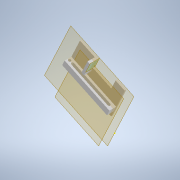
# Autodesk Inventor part: s_support_bottom
Saved by Autodesk Inventor 2020.1 (Build 241239000, 239)
## iProperties
Created: 2019-10-17
Part Number: s_support_bottom
Material: Generic
Document SubType Name: Modeling
Designer: jesse
Density: 1 g/cm^3
Appearance: Default
support_length: 2.300 in
hole_size: 0.118 in
Author: jesse
Autodesk Inventor part; units mm, degrees
ref_plane "YZ Plane" through (0, 0, 0) normal (1, 0, 0) x (0, 1, 0)
ref_plane "XZ Plane" through (0, 0, 0) normal (0, 1, 0) x (-1, 0, 0)
ref_plane "XY Plane" through (0, 0, 0) normal (0, 0, 1) x (1, 0, 0)
ref_plane "Work Plane1" through (19.722, 36.341, 0) normal (0, 0, 1) x (0.4250843, 0.9051538, 0)
sketch "Sketch1" plane through (19.722, 36.341, 0) normal (0, 0, 1) x (0.4250843, 0.9051538, 0)
  line L0 (-12.1227, 70.1452) -> (-18.8796, 70.1452)
  line L1 (-18.8796, 70.1452) -> (-18.8796, 11.7252)
  line L2 (-18.8796, 11.7252) -> (-12.1227, 11.7252)
  line L3 (-12.1227, 11.7252) -> (-12.1227, 70.1452)
  point P0 (-41.2777, 2.4034)
  dimension "support_length" = 58.42
  constraints: 8 end point, 2 parallel, 1 horizontal, 1 perpendicular
  measures "support_length" distance of L2.end L0.start
extrude "Extrusion1" add sketch "Sketch1" along normal blind 8
sketch "Sketch2" plane through (1.0834, 24.2363, 0) normal (-0.4250843, -0.9051538, 0) x (0, 0, 1)
  line L0 (0, 58.42) -> (8, 58.42) construction
  line L1 (4, 58.42) -> (4, 0) construction
  line L2 (0, 0) -> (8, 0) construction
  line L3 (4, 52.42) -> (4, 5) construction
  line L4 (2.5, 52.42) -> (2.5, 5)
  line L5 (5.5, 5) -> (5.5, 52.42)
  arc A0 (5.5, 52.42) -> (2.5, 52.42) centre (4, 52.42) ccw
  arc A1 (2.5, 5) -> (5.5, 5) centre (4, 5) ccw
  line L6 (4, 5) -> (6.3728, 5) construction
  line L7 (4, 52.42) -> (6.6371, 52.42) construction
  line L8 (5.634, 5) -> (5.634, 0) construction
  circle A2 centre (4, 56.42) radius 1.5
  line L9 (4, 56.42) -> (7.1435, 56.42) construction
  point P0 (0, -9.3218)
  point P1 (4, 28.71)
  dimension "d5" = 3
  dimension "d6" = 3
  dimension "d7" = 2
  dimension "d8" = 5
  dimension "d9" = 4
  constraints: 18 end point, 5 point on line, 4 point on circle, 4 tangent, 3 centre point, 3 horizontal, 3 midpoint, 1 parallel
  measures "d5" distance between parallel lines of L4 L5
  measures "d6" diameter of A2
  measures "d7" distance between parallel lines of L9 L0
  measures "d8" distance between parallel lines of L6 L2
  measures "d9" distance between parallel lines of L7 L9
extrude "Extrusion2" cut sketch "Sketch2" against normal blind 15.875
sketch "Sketch3" plane through (19.722, 36.341, 0) normal (0, 0, -1) x (-0.9051538, 0.4250843, 0)
  line L0 (70.1452, -12.1227) -> (70.1452, -18.8796) construction
  line L1 (11.7252, -12.1227) -> (70.1452, -12.1227) construction
  line L2 (70.1452, -18.8796) -> (11.7252, -12.1227) construction
  line L3 (70.1452, -4.7378) -> (11.7252, -4.7378)
  line L4 (11.7252, -4.7378) -> (11.7252, -26.2645)
  line L5 (11.7252, -26.2645) -> (70.1452, -26.2645)
  line L6 (70.1452, -26.2645) -> (70.1452, -4.7378)
  line L7 (70.1452, -4.7378) -> (11.7252, -26.2645) construction
  line L8 (11.7252, -4.7378) -> (70.1452, -26.2645) construction
  line L9 (11.7252, -18.8796) -> (11.7252, -12.1227) projected
  point P0 (2.4034, -41.2777)
  point P1 (40.9352, -15.5011)
  constraints: 14 end point, 3 midpoint, 2 parallel, 1 collinear, 1 horizontal, 1 perpendicular
extrude "Extrusion3" add sketch "Sketch3" along normal blind 2
ref_plane "Work Plane2" through (-46.3647, 46.5192, 4) normal (0, 0, 1) x (0.9051538, -0.4250843, 0)
sketch "Sketch4" plane through (19.722, 36.341, -2) normal (0, 0, -1) x (-0.9051538, 0.4250843, 0)
  point P0 (2.4034, -41.2777)
ref_plane "Work Plane3" through (-28.5317, 57.7215, 3) normal (-0.9051538, 0.4250843, 0) x (-0.4250843, -0.9051538, 0)
sketch "Sketch5" plane through (-28.5317, 57.7215, 3) normal (-0.9051538, 0.4250843, 0) x (-0.4250843, -0.9051538, 0)
  line L0 (3.5785, -5) -> (25.1052, -5) projected
  line L1 (-12.9356, 5.5866) -> (3.721, 5.5866)
  line L2 (3.721, 5.5866) -> (3.721, -5)
  line L3 (3.721, -5) -> (-12.9356, -5)
  line L4 (-12.9356, -5) -> (-12.9356, 5.5866)
  line L5 (-12.9356, -4) -> (-12.9356, 4) projected
  point P0 (40.1184, -3)
  constraints: 8 end point, 2 parallel, 1 collinear, 1 horizontal, 1 perpendicular, 1 point on line
extrude "Extrusion4" add sketch "Sketch5" along normal blind 3.175
sketch "Sketch6" plane through (-45.7842, 61.8702, 0) normal (0.4250843, 0.9051538, 0) x (0.9051538, -0.4250843, 0)
  line L0 (14.2048, 0) -> (14.2048, 2) projected
  line L1 (0, 2) -> (14.2048, 2) projected
  line L2 (0, 0) -> (0, 2) projected
  line L3 (0, 0) -> (14.2048, 0) projected
  line L4 (17.3798, 2) -> (17.3798, 0) projected
  line L5 (17.3798, 0) -> (58.42, 0) projected
  line L6 (58.42, 0) -> (58.42, 2) projected
  line L7 (17.3798, 2) -> (58.42, 2) projected
  point P0 (67.7418, 0)
ref_plane "Work Plane4" through (-19.2599, 54.4009, -1.0016) normal (-0.4250843, -0.9051538, 0) x (0.9051538, -0.4250843, 0)
extrude "Extrusion5" add sketch "Sketch6" along normal up to surface (4.5142 mm away)
sketch "Sketch7" plane through (-31.0078, 59.918, 0) normal (0.4250843, 0.9051538, 0) x (0.9051538, -0.4250843, 0)
  line L0 (0, 2) -> (0, 0) projected
  line L1 (0, 2) -> (-14.2048, 2) projected
  line L2 (-14.2048, 2) -> (-14.2048, 0) projected
  line L3 (-14.2048, 0) -> (0, 0) projected
  point P0 (53.537, 0)
extrude "Extrusion6" add sketch "Sketch7" along normal up to surface (12 mm away)
sketch "Sketch8" plane through (9.0138, 41.1228, 0) normal (0.4250843, 0.9051538, 0) x (0.9051538, -0.4250843, 0)
  line L0 (-17.0402, -2.3011) -> (-17.0402, 1.6) projected
  line L1 (0, 0) -> (-58.42, 0) projected
  line L2 (0, 2) -> (-41.0402, 2) projected
  line L3 (-17.0402, 0) -> (0, 0)
  line L4 (0, 0) -> (0, 2)
  line L5 (0, 2) -> (-17.0402, 2)
  line L6 (-17.0402, 2) -> (-17.0402, 0)
  point P0 (9.3218, 0)
  point P1 (0, 0)
  point P2 (-17.0402, 2)
  constraints: 8 end point, 2 parallel, 2 point on line, 1 horizontal, 1 perpendicular
extrude "Extrusion7" add sketch "Sketch8" along normal up to surface (12 mm away)
sketch "Sketch9" plane through (-31.4055, 59.0711, 3) normal (-0.9051538, 0.4250843, 0) x (0, 0, 1)
  arc A0 (-1.2091, 7.8234) -> (1.0166, 8.0386) centre (0, 6.9356) ccw construction
  line L0 (-1.2091, 7.8234) -> (1.0166, 8.0386) construction
  circle A1 centre (0, 6.9356) radius 2
  circle A2 centre (0, 11.4356) radius 0.625 projected
  circle A3 centre (0, 2.4356) radius 0.625 projected
  point P0 (-3, -40.1184)
  dimension "d20" = 0.5
  constraints: 1 centre point, 1 coincident
  measures "d20" radial gap between concentric circles of A0 A1
extrude "Extrusion8" cut sketch "Sketch9" against normal through all
fillet "Fillet1" radius 3.175 1 edges at (-29.1237, 56.4609, 0)
sketch "Sketch10" plane through (19.722, 36.341, 0) normal (0, 0, 1) x (0.9051538, -0.4250843, 0)
  line L0 (-75.2252, 16.2156) -> (-75.2252, 4.5316) projected
  arc A0 (-68.6212, 11.1356) -> (-75.2252, 4.5316) centre (-68.6212, 4.5316) ccw construction
  line L1 (-67.6052, 11.1356) -> (-68.6212, 11.1356) projected
  line L2 (-67.6052, 11.1356) -> (-67.6052, 15.9616) projected
  arc A1 (-61.0012, 22.5656) -> (-67.6052, 15.9616) centre (-61.0012, 15.9616) ccw projected
  line L3 (-61.0012, 22.5656) -> (-68.8752, 22.5656) projected
  arc A2 (-68.8752, 22.5656) -> (-75.2252, 16.2156) centre (-68.8752, 16.2156) ccw projected
  circle A3 centre (-71.4152, 16.2156) radius 1.1303 construction
  arc A4 (-68.6212, 11.1356) -> (-75.2252, 4.5316) centre (-68.6212, 4.5316) ccw construction
  line L4 (-75.2252, 4.5316) -> (-75.2252, 1.2354) projected
  line L5 (-75.2252, 1.2354) -> (-67.6052, 1.2354) projected
  line L6 (-67.6052, 1.2354) -> (-67.6052, 11.1356) projected
  line L7 (-67.6052, 11.1356) -> (-68.6212, 11.1356) projected
  circle A5 centre (-71.4152, 6.0556) radius 1.1303 construction
  line L8 (-11.7252, -3.0884) -> (-11.7252, 4.5316) projected
  arc A6 (-11.7252, 4.5316) -> (-18.3292, 11.1356) centre (-18.3292, 4.5316) ccw construction
  line L9 (-18.3292, 11.1356) -> (-19.3452, 11.1356) projected
  line L10 (-19.3452, 3.5156) -> (-19.3452, 11.1356) projected
  line L11 (-18.3292, 3.5156) -> (-19.3452, 3.5156) projected
  arc A7 (-11.7252, -3.0884) -> (-18.3292, 3.5156) centre (-18.3292, -3.0884) ccw projected
  circle A8 centre (-15.5352, 6.0556) radius 1.1303 construction
  line L12 (-18.3292, 11.1356) -> (-19.3452, 11.1356) construction
  arc A9 (-11.7252, 4.5316) -> (-18.3292, 11.1356) centre (-18.3292, 4.5316) ccw construction
  line L13 (-11.7252, 4.5316) -> (-11.7252, 16.2156) projected
  arc A10 (-11.7252, 16.2156) -> (-18.0752, 22.5656) centre (-18.0752, 16.2156) ccw projected
  line L14 (-18.0752, 22.5656) -> (-25.9492, 22.5656) projected
  arc A11 (-19.3452, 15.9616) -> (-25.9492, 22.5656) centre (-25.9492, 15.9616) ccw projected
  line L15 (-19.3452, 15.9616) -> (-19.3452, 11.1356) projected
  circle A12 centre (-15.5352, 16.2156) radius 1.1303 construction
  point P0 (-2.4034, -41.2777)
extrude "Extrusion9" cut sketch "Sketch10" against normal blind 26.9875
sketch "Sketch11" plane through (19.722, 36.341, 0) normal (0, 0, 1) x (0.9051538, -0.4250843, 0)
  line L0 (-19.4861, 3.5156) -> (-18.3292, 3.5156) projected
  ellipse E0 centre (-25.9492, 1.597) end of major axis (-25.9492, 10.9364) minor radius 6.604 (-19.4861, 3.5156) -> (-25.9492, 10.9364) ccw projected
  line L1 (-25.9492, 10.9364) -> (-61.0012, 10.9364) projected
  ellipse E1 centre (-61.0012, 1.597) end of major axis (-61.0012, -7.7425) minor radius 6.604 (-61.0012, 10.9364) -> (-67.4644, 3.5156) ccw projected
  line L2 (-68.6212, 3.5156) -> (-67.4644, 3.5156) projected
  arc A0 (-68.6212, 3.5156) -> (-75.2252, -3.0884) centre (-68.6212, -3.0884) ccw projected
  line L3 (-75.2252, -3.0884) -> (-75.2252, -15.2804) projected
  arc A1 (-75.2252, -15.2804) -> (-68.6212, -21.8844) centre (-68.6212, -15.2804) ccw projected
  line L4 (-67.6052, -21.8844) -> (-68.6212, -21.8844) projected
  line L5 (-67.6052, -34.3304) -> (-67.6052, -21.8844) projected
  arc A2 (-67.6052, -34.3304) -> (-61.0012, -40.9344) centre (-61.0012, -34.3304) ccw projected
  line L6 (-61.0012, -40.9344) -> (-25.9492, -40.9344) projected
  arc A3 (-25.9492, -40.9344) -> (-19.3452, -34.3304) centre (-25.9492, -34.3304) ccw projected
  line L7 (-19.3452, -21.8844) -> (-19.3452, -34.3304) projected
  line L8 (-18.3292, -21.8844) -> (-19.3452, -21.8844) projected
  arc A4 (-18.3292, -21.8844) -> (-11.7252, -15.2804) centre (-18.3292, -15.2804) ccw projected
  line L9 (-11.7252, -3.0884) -> (-11.7252, -15.2804) projected
  arc A5 (-11.7252, -3.0884) -> (-18.3292, 3.5156) centre (-18.3292, -3.0884) ccw projected
  line L10 (3.3894, -48.6509) -> (-95.174, -48.6509)
  line L11 (-95.174, -48.6509) -> (-95.174, 27.8086)
  line L12 (-95.174, 27.8086) -> (3.3894, 27.8086)
  line L13 (3.3894, 27.8086) -> (3.3894, -48.6509)
  point P0 (-2.4034, -41.2777)
  constraints: 8 end point, 2 parallel, 1 horizontal, 1 perpendicular, 2 other
extrude "Extrusion10" cut sketch "Sketch11" against normal through all both and the other way through all
equation "\"d5\" = hole_size"
equation "\"d6\" = hole_size"
equation "\"hole_size\" = 3"
body "Solid1"
